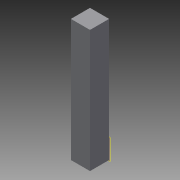
# Autodesk Inventor part: front peice left
Saved by Autodesk Inventor 2015 (Build 190159000, 159)
## iProperties
Created: 2014-10-04
Part Number: front peice left
Material: Generic
Document SubType Name: Modeling
Designer: jesse
Density: 1 g/cm^3
Appearance: Default
Author: jesse
Autodesk Inventor part; units mm, degrees
ref_plane "YZ Plane" through (0, 0, 0) normal (1, 0, 0) x (0, 1, 0)
ref_plane "XZ Plane" through (0, 0, 0) normal (0, 1, 0) x (-1, 0, 0)
ref_plane "XY Plane" through (0, 0, 0) normal (0, 0, 1) x (1, 0, 0)
ref_plane "Work Plane1" through (0, -116.2633, 0) normal (0, 0, 1) x (1, 0, 0)
sketch "Sketch1" plane through (0, -116.2633, 0) normal (0, 0, 1) x (1, 0, 0)
  line L0 (-9.525, -9.525) -> (9.525, -9.525) projected
  line L1 (9.525, 82.804) -> (-9.525, 82.804) projected
  line L2 (-9.525, 82.804) -> (-9.525, -9.525)
  line L3 (9.525, -9.525) -> (9.525, 82.804)
  point P0 (0, 116.2633)
  constraints: 4 end point, 1 parallel, 1 perpendicular
extrude "Extrusion1" add sketch "Sketch1" along normal blind 19.05
body "Solid1"
